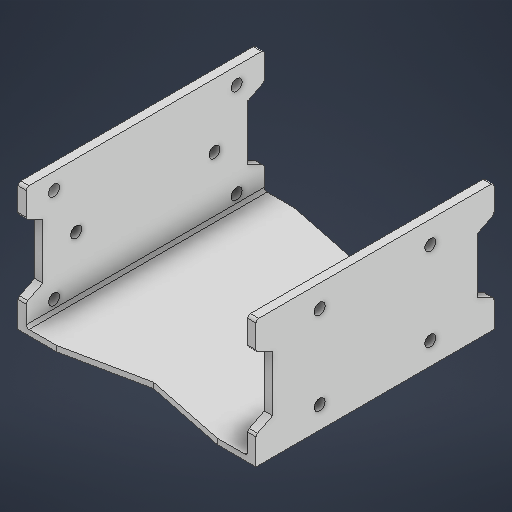
# Autodesk Inventor part: BiaFrame
Saved by Autodesk Inventor 2027 (Build 310192060, 192F)
## iProperties
Created: 2026-09-09
Part Number: BiaFrame
Material: Genérico
Document SubType Name: Modeling
Designer: paulo
Density: 1 g/cm^3
Appearance: Padrão
Author: paulo
Autodesk Inventor part; units mm, degrees
ref_plane "YZ Plane" through (0, 0, 0) normal (1, 0, 0) x (0, 1, 0)
ref_plane "XZ Plane" through (0, 0, 0) normal (0, 1, 0) x (-1, 0, 0)
ref_plane "XY Plane" through (0, 0, 0) normal (0, 0, 1) x (1, 0, 0)
sketch "Esboço1" plane through (0, 0, 0) normal (0, 1, 0) x (-1, 0, 0)
  line L0 (-21.5, 21.5) -> (-21.5, -21.5)
  line L1 (21.5, -21.5) -> (21.5, 21.5)
  line L2 (21.5, 21.5) -> (-21.5, -21.5) construction
  line L3 (-21.5, 21.5) -> (21.5, -21.5) construction
  line L4 (21.5, -21.5) -> (14.5, -21.5)
  line L5 (14.5, -21.5) -> (0, -18.5)
  line L6 (-21.5, -21.5) -> (-14.5, -21.5)
  line L7 (-14.5, -21.5) -> (0, -18.5)
  line L8 (-21.5, -21.5) -> (-14.5, -21.5)
  line L9 (14.5, -21.5) -> (21.5, -21.5)
  line L10 (21.5, 21.5) -> (14.5, 21.5)
  line L11 (14.5, 21.5) -> (0, 18.5)
  line L12 (-21.5, 21.5) -> (-14.5, 21.5)
  line L13 (-14.5, 21.5) -> (0, 18.5)
  line L14 (20, -20) -> (20, 20)
  line L15 (20, 20) -> (14.6535, 20)
  line L16 (14.6535, 20) -> (0, 16.9682)
  line L17 (0, 16.9682) -> (-14.6535, 20)
  line L18 (-14.6535, 20) -> (-20, 20)
  line L19 (-20, 20) -> (-20, -20)
  line L20 (20, -20) -> (14.6535, -20)
  line L21 (14.6535, -20) -> (0, -16.9682)
  line L22 (0, -16.9682) -> (-14.6535, -20)
  line L23 (-14.6535, -20) -> (-20, -20)
  line L24 (20, 20) -> (20, 21.5)
  line L25 (20, -20) -> (20, -21.5)
  line L26 (-20, -20) -> (-20, -21.5)
  line L27 (-20, 20) -> (-20, 21.5)
  point P0 (0, 0)
  dimension "d0" = 43
  dimension "d1" = 43
  dimension "d2" = 37
  dimension "d3" = 7
  dimension "d4" = 7
  constraints: 56 end point, 7 point on line, 3 perpendicular, 2 midpoint, 2 parallel, 1 vertical, 4 other
  measures "d0" distance of L1.start L0.end
  measures "d1" distance of L0.end L0.start
  measures "d2" distance of L11.end L5.end
  measures "d3" distance of L1.start L4.end
  measures "d4" distance of L0.end L6.end
extrude "Extrusão1" add sketch "Esboço1" along normal blind 23 contours L12 L27 L19 L26 L6 L0 | L10 L1 L4 L25 L14 L24
extrude "Extrusão2" add sketch "Esboço1" along normal blind 1 contours L12 L13 L11 L10 L24 L15 L16 L17 L18 L27 | L26 L23 L22 L21 L20 L25 L4 L5 L7 L6 | L18 L17 L16 L15 L14 L20 L21 L22 L23 L19
sketch "Esboço2" plane through (-21.5, 0, -21.5) normal (-1, 0, 0) x (0, 0, 1)
  line L0 (0, 0) -> (0, 23) projected
  line L1 (0, 23) -> (0, 18)
  line L2 (3, 0) -> (0, 0) projected
  line L3 (0, 0) -> (0, 5)
  line L4 (0, 11.5) -> (43, 11.5)
  line L5 (43, 0) -> (43, 23) projected
  line L6 (3, 11.5) -> (40, 11.5)
  line L7 (3, 16.5) -> (3, 6.5)
  line L8 (0, 18) -> (3, 16.5)
  line L9 (0, 5) -> (3, 6.5)
  line L10 (0, 18) -> (0, 5)
  line L11 (43, 23) -> (0, 23) projected
  line L12 (21.5, 23) -> (21.5, 0)
  line L13 (43, 23) -> (43, 18)
  line L14 (43, 0) -> (43, 5)
  line L15 (40, 16.5) -> (40, 6.5)
  line L16 (43, 18) -> (40, 16.5)
  line L17 (43, 5) -> (40, 6.5)
  line L18 (43, 18) -> (43, 5)
  line L19 (43, 0) -> (0, 0) projected
  line L20 (43, 0) -> (38, 0)
  line L21 (43, 5) -> (43, 0)
  circle A0 centre (38, 3) radius 1
  circle A1 centre (38, 20) radius 1
  circle A2 centre (5, 3) radius 1
  circle A3 centre (5, 20) radius 1
  line L22 (0, 11.5) -> (8, 11.5)
  line L23 (8, 11.5) -> (9, 11.5)
  circle A4 centre (9, 11.5) radius 1
  line L24 (43, 11.5) -> (34, 11.5)
  circle A5 centre (34, 11.5) radius 1
  point P0 (21.5, 11.5)
  dimension "d15" = 5
  dimension "d16" = 5
  dimension "d17" = 37
  dimension "d18" = 10
  dimension "d26" = 2
  dimension "d29" = 17
  dimension "d32" = 33
  dimension "d35" = 8
  dimension "d36" = 1
  dimension "d37" = 2
  dimension "d38" = 3
  dimension "d39" = 5
  dimension "d40" = 9
  dimension "d41" = 2
  constraints: 40 end point, 6 centre point, 6 midpoint, 6 point on line, 4 symmetric about line, 3 vertical, 2 coincident, 2 horizontal, 1 collinear, 6 other
  measures "d15" distance of L0.end L1.end
  measures "d16" distance of L0.start L3.end
  measures "d17" distance of L6.start L6.end
  measures "d18" distance of L7.start L7.end
  measures "d26" diameter of A0
  measures "d29" distance of A0.centre A1.centre
  measures "d32" distance of A0.centre A2.centre
  measures "d35" distance of L4.start L22.end
  measures "d36" distance of L22.end L23.end
  measures "d37" diameter of A4
  measures "d38" distance from line of L19 A0.centre
  measures "d39" distance from line of L5 A0.centre
  measures "d40" distance of L4.end L24.end
  measures "d41" diameter of A5
extrude "Extrusão3" cut sketch "Esboço2" along normal blind 1 and the other way blind 60.75 contours L0 L4 L7 L9 | L0 L8 L7 L4 | L17 L15 L4 L5 | L15 L16 L5 L4
extrude "Extrusão4" cut sketch "Esboço2" against normal blind 3 contours A4 L4 | L4 A4 | A5 L4 | L4 A5 | A0 | A1 | A2 | A3
sketch "Esboço5" plane through (21.5, 0, 21.5) normal (1, 0, 0) x (0, 0, -1)
  line L0 (11.5, 0) -> (31.5, 0)
  line L1 (0, 0) -> (43, 0) projected
  line L2 (11.5, 0) -> (11.5, 4)
  line L3 (31.5, 0) -> (31.5, 3)
  circle A0 centre (11.5, 4) radius 1
  circle A1 centre (31.5, 4) radius 1
  circle A2 centre (11.5, 19) radius 1
  circle A3 centre (31.5, 19) radius 1
  line L4 (0, 23) -> (43, 23) projected
  point P0 (21.5, 0)
  dimension "d46" = 3
  dimension "d47" = 2
  dimension "d50" = 20
  dimension "d53" = 15
  dimension "d56" = 4
  constraints: 6 end point, 4 centre point, 3 vertical, 1 coincident, 1 horizontal, 1 midpoint, 1 point on line, 6 other
  measures "d46" distance of L0.end L3.end
  measures "d47" diameter of A0
  measures "d50" distance of A0.centre A1.centre
  measures "d53" distance of A0.centre A2.centre
  measures "d56" distance from line of L4 A3.centre
extrude "Extrusão5" cut sketch "Esboço5" against normal blind 3
fillet "Arredondamento2" radius 0.5 14 edges at (-20, 1, 0) (20, 1, 0) (-20.75, 23, -21.5) (-20.75, 18, -21.5) (-20.75, 5, -21.5) (20.75, 5, -21.5) (20.75, 18, -21.5) (20.75, 23, -21.5) (20.75, 23, 21.5) (20.75, 18, 21.5) (20.75, 5, 21.5) (-20.75, 5, 21.5) (-20.75, 18, 21.5) (-20.75, 23, 21.5)
